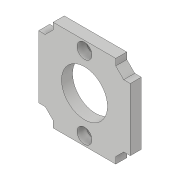
# Autodesk Inventor part: 20_Cube_insert_Sample_holder_v3
Saved by Autodesk Inventor 2022 (Build 260153000, 153)
## iProperties
Created: 2019-08-07
Part Number: 20_Cube_insert_Sample_holder_v3
Material: Generic
Document SubType Name: Modeling
Designer: marsikovabarbora
Density: 1 g/cm^3
Appearance: Default
Catalog Web Link: isPrinted
Vendor: openUC2
Author: marsikovabarbora
Autodesk Inventor part; units mm, degrees
ref_plane "YZ Plane" through (0, 0, 0) normal (1, 0, 0) x (0, 1, 0)
ref_plane "XZ Plane" through (0, 0, 0) normal (0, 1, 0) x (-1, 0, 0)
ref_plane "XY Plane" through (0, 0, 0) normal (0, 0, 1) x (1, 0, 0)
sketch "Sketch1" plane through (0, 0, 0) normal (0, 0, 1) x (1, 0, 0)
  line L0 (-34.86, 0) -> (34.86, 0) construction
  line L1 (0, -34.86) -> (0, 34.86) construction
  line L2 (0, 0) -> (11.157509, 11.157509) construction
  line L3 (0, 0) -> (15.7791, 0) construction
  line L4 (0, 24.9) -> (16.800857, 24.9)
  line L5 (16.800857, 24.9) -> (16.800857, 21.241488)
  line L6 (16.800857, 21.241488) -> (19.021172, 19.021172)
  line L7 (24.9, 0) -> (24.9, 16.800857)
  line L8 (24.9, 16.800857) -> (21.241488, 16.800857)
  line L9 (21.241488, 16.800857) -> (19.021172, 19.021172)
  line L10 (0, -24.9) -> (16.800857, -24.9)
  line L11 (16.800857, -24.9) -> (16.800857, -21.241488)
  line L12 (16.800857, -21.241488) -> (19.021172, -19.021172)
  line L13 (24.9, 0) -> (24.9, -16.800857)
  line L14 (24.9, -16.800857) -> (21.241488, -16.800857)
  line L15 (21.241488, -16.800857) -> (19.021172, -19.021172)
  line L16 (0, 24.9) -> (-16.800857, 24.9)
  line L17 (-16.800857, 24.9) -> (-16.800857, 21.241488)
  line L18 (-16.800857, 21.241488) -> (-19.021172, 19.021172)
  line L19 (-24.9, 16.800857) -> (-21.241488, 16.800857)
  line L20 (-21.241488, 16.800857) -> (-19.021172, 19.021172)
  line L21 (0, -24.9) -> (-16.800857, -24.9)
  line L22 (-16.800857, -24.9) -> (-16.800857, -21.241488)
  line L23 (-16.800857, -21.241488) -> (-19.021172, -19.021172)
  line L24 (-21.241488, -16.800857) -> (-19.021172, -19.021172)
  line L25 (-24.9, -16.800857) -> (-21.241488, -16.800857)
  line L26 (-24.9, 0) -> (-24.9, -16.800857)
  line L27 (-24.9, 0) -> (-24.9, 16.800857)
  circle A0 centre (0, 0) radius 12.5
  dimension "d0" = 45
  dimension "d2" = 24.9
  dimension "d3" = 3.14
  dimension "d4" = 26.9
  dimension "d5" = 25
  constraints: 52 end point, 20 symmetric about line, 2 horizontal, 2 perpendicular, 2 point on line, 1 centre point, 1 coincident, 1 equal length
  measures "d0" angle of L3 L2
  measures "d2" distance between parallel lines of L0 L4
  measures "d3" distance of L5.end L6.end
  measures "d4" distance from line of L2.start L6
  measures "d5" diameter of A0
extrude "Extrusion1" add sketch "Sketch1" along normal blind 6
sketch "Sketch4" plane through (0, 0, 0) normal (0, 0, -1) x (-1, 0, 0)
  circle A0 centre (0, 0) radius 12.5 construction
  line L0 (16.800857, 24.9) -> (-16.800857, 24.9) construction
  line L1 (-16.800857, 24.9) -> (-16.800857, 21.241488)
  line L2 (-16.800857, 21.241488) -> (-21.241488, 16.800857)
  line L3 (-21.241488, 16.800857) -> (-24.9, 16.800857)
  line L4 (-24.9, 16.800857) -> (-24.9, -16.800857) construction
  line L5 (-24.9, -16.800857) -> (-21.241488, -16.800857)
  line L6 (-21.241488, -16.800857) -> (-16.800857, -21.241488)
  line L7 (-16.800857, -21.241488) -> (-16.800857, -24.9)
  line L8 (-16.800857, -24.9) -> (16.800857, -24.9) construction
  line L9 (16.800857, -24.9) -> (16.800857, -21.241488)
  line L10 (16.800857, -21.241488) -> (21.241488, -16.800857)
  line L11 (21.241488, -16.800857) -> (24.9, -16.800857)
  line L12 (24.9, -16.800857) -> (24.9, 16.800857) construction
  line L13 (24.9, 16.800857) -> (21.241488, 16.800857)
  line L14 (21.241488, 16.800857) -> (16.800857, 21.241488)
  line L15 (16.800857, 21.241488) -> (16.800857, 24.9)
  line L16 (-17.000857, 25.1) -> (17.000857, 25.1) construction
  line L17 (17.000857, 25.1) -> (17.000857, 21.32433)
  line L18 (17.000857, 21.32433) -> (21.32433, 17.000857)
  line L19 (21.32433, 17.000857) -> (25.1, 17.000857)
  line L20 (25.1, 17.000857) -> (25.1, -17.000857) construction
  line L21 (25.1, -17.000857) -> (21.32433, -17.000857)
  line L22 (21.32433, -17.000857) -> (17.000857, -21.32433)
  line L23 (17.000857, -21.32433) -> (17.000857, -25.1)
  line L24 (17.000857, -25.1) -> (-17.000857, -25.1) construction
  line L25 (-17.000857, -25.1) -> (-17.000857, -21.32433)
  line L26 (-17.000857, -21.32433) -> (-21.32433, -17.000857)
  line L27 (-21.32433, -17.000857) -> (-25.1, -17.000857)
  line L28 (-25.1, -17.000857) -> (-25.1, 17.000857) construction
  line L29 (-25.1, 17.000857) -> (-21.32433, 17.000857)
  line L30 (-21.32433, 17.000857) -> (-17.000857, 21.32433)
  line L31 (-17.000857, 21.32433) -> (-17.000857, 25.1)
  line L32 (-24.9, -16.800857) -> (-24.9, 16.800857)
  line L33 (-24.9, 16.800857) -> (-24.9, 17.000857)
  line L34 (-16.800857, 24.9) -> (-17.000857, 24.9)
  line L35 (-16.800857, 24.9) -> (16.800857, 24.9)
  line L36 (16.800857, 24.9) -> (17.000857, 24.9)
  line L37 (24.9, 16.800857) -> (24.9, 17.000857)
  line L38 (24.9, 16.800857) -> (24.9, -16.800857)
  line L39 (24.9, -16.800857) -> (24.9, -17.000857)
  line L40 (16.800857, -24.9) -> (-16.800857, -24.9)
  line L41 (16.800857, -24.9) -> (17.000857, -24.9)
  line L42 (-16.800857, -24.9) -> (-17.000857, -24.9)
  line L43 (-24.9, -16.800857) -> (-24.9, -17.000857)
  dimension "d19" = 0.2
  constraints: 48 end point, 12 point on line, 4 perpendicular, 15 other
  measures "d19" distance between parallel lines of L0 L16
extrude "IM_offset" add sketch "Sketch4" against normal up to surface (6 mm away) contours L1 L2 L3 L33 L29 L30 L31 L34 | L36 L17 L18 L19 L37 L13 L14 L15 | L5 L6 L7 L42 L25 L26 L27 L43 | L39 L21 L22 L23 L41 L9 L10 L11
sketch "Skizze5" plane through (0, 0, 6) normal (0, 0, 1) x (1, 0, 0)
  circle A0 centre (0, 0) radius 12.5
  line L0 (-17.000857, 24.9) -> (17.000857, 24.9)
  line L1 (-17.000857, 21.32433) -> (-17.000857, 24.9)
  line L2 (-21.32433, 17.000857) -> (-17.000857, 21.32433)
  line L3 (-24.9, 17.000857) -> (-21.32433, 17.000857)
  line L4 (-24.9, -17.000857) -> (-24.9, 17.000857)
  line L5 (-21.32433, -17.000857) -> (-24.9, -17.000857)
  line L6 (-17.000857, -21.32433) -> (-21.32433, -17.000857)
  line L7 (-17.000857, -24.9) -> (-17.000857, -21.32433)
  line L8 (17.000857, -24.9) -> (-17.000857, -24.9)
  line L9 (17.000857, -21.32433) -> (17.000857, -24.9)
  line L10 (21.32433, -17.000857) -> (17.000857, -21.32433)
  line L11 (24.9, -17.000857) -> (21.32433, -17.000857)
  line L12 (24.9, 17.000857) -> (24.9, -17.000857)
  line L13 (21.32433, 17.000857) -> (24.9, 17.000857)
  line L14 (17.000857, 21.32433) -> (21.32433, 17.000857)
  line L15 (17.000857, 24.9) -> (17.000857, 21.32433)
  circle A1 centre (0, 0) radius 20
  circle A2 centre (0, 20) radius 4.05
  circle A3 centre (0, -20) radius 4.05
  dimension "d22" = 40
  dimension "d23" = 8.1
  dimension "d24" = 8.1
  constraints: 3 centre point, 2 point on circle, 1 coincident
  measures "d22" diameter of A1
  measures "d23" diameter of A2
  measures "d24" diameter of A3
sketch "Skizze5 outline for Extrusion4" plane through (0, 0, 6) normal (0, 0, 1) x (1, 0, 0)
  circle A0 centre (0, -20) radius 4.05
  circle A1 centre (0, 20) radius 4.05
extrude "Extrusion4" cut sketch "Skizze5 outline for Extrusion4" against normal blind 5 draft -1
body "Solid1"
